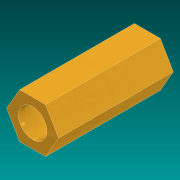
# Autodesk Inventor part: spacerHex
Saved by Autodesk Inventor 2020.3 (Build 243373000, 373)
## iProperties
Created: 2020-05-27
Part Number: spacerHex
Material: Brass, Soft Yellow, Welded
Document SubType Name: Modeling
Designer: Svend
Density: 8.5 g/cm^3
Appearance: Weld - Brass
Author: Svend
Autodesk Inventor part; units mm, degrees
ref_plane "YZ Plane" through (0, 0, 0) normal (1, 0, 0) x (0, 1, 0)
ref_plane "XZ Plane" through (0, 0, 0) normal (0, 1, 0) x (-1, 0, 0)
ref_plane "XY Plane" through (0, 0, 0) normal (0, 0, 1) x (1, 0, 0)
sketch "Sketch1" plane through (0, 0, 0) normal (0, 0, 1) x (1, 0, 0)
  line L0 (1.3568, 2.35) -> (2.7135, 0)
  line L1 (2.7135, 0) -> (1.3568, -2.35)
  line L2 (1.3568, -2.35) -> (-1.3568, -2.35)
  line L3 (-1.3568, -2.35) -> (-2.7135, 0)
  line L4 (-2.7135, 0) -> (-1.3568, 2.35)
  line L5 (-1.3568, 2.35) -> (1.3568, 2.35)
  circle A0 centre (0, 0) radius 1.5
  point P0 (0, 2.35)
  dimension "d0" = 4.7
  dimension "d1" = 3
  constraints: 12 end point, 2 coincident, 1 centre point, 1 midpoint, 1 vertical alignment, 13 other
  measures "d0" distance between parallel lines of L2 L5
  measures "d1" diameter of A0
extrude "Extrusion1" add sketch "Sketch1" along normal mid plane 12
body "Solid1"
